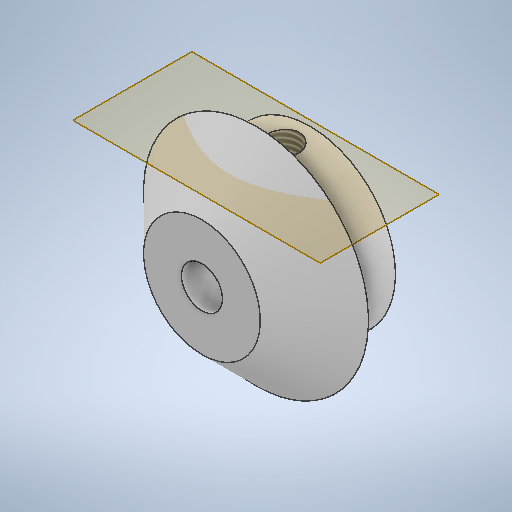
# Autodesk Inventor part: guide
Saved by Autodesk Inventor 2025.1 (Build 291241000, 241)
## iProperties
Created: 2025-03-11
Part Number: guide
Material: Generic
Document SubType Name: Modeling
Designer: santiago
Density: 1 g/cm^3
Appearance: Default
Author: santiago
Autodesk Inventor part; units mm, degrees
ref_plane "YZ Plane" through (0, 0, 0) normal (1, 0, 0) x (0, 1, 0)
ref_plane "XY Plane" through (0, 0, 0) normal (0, 0, 1) x (1, 0, 0)
sketch "Sketch1" plane through (0, 0, 0) normal (1, 0, 0) x (0, 1, 0)
  line L0 (0.0289, 5.9359) -> (3.5289, 5.9359)
  line L1 (0.0289, 5.9359) -> (0.0289, -4.0641)
  line L2 (-1.8711, 5.9359) -> (-1.8711, -4.0641) construction
  line L3 (6.0289, 0.9359) -> (8.5289, 0.9359)
  line L4 (3.5289, 5.9359) -> (8.5289, 0.9359)
  line L5 (0.0289, -4.0641) -> (6.0289, -4.0641)
  line L6 (6.0289, -4.0641) -> (6.0289, 0.9359)
  point P0 (0, 0)
  dimension "d0" = 3.5
  dimension "d3" = 10
  dimension "d4" = 1.9
  constraints: 14 end point, 3 horizontal, 2 vertical, 1 perpendicular
  measures "d0" distance of L0.start L0.end
  measures "d3" distance of L0.start L1.end
  measures "d4" distance between parallel lines of L1 L2
revolve "Revolution1" add sketch "Sketch1" angle 360 about axis through (0, -1.8711, 5.9359) along (0, 0, -1)
ref_plane "Work Plane1" through (0, 6.0289, -1.5641) normal (0, 1, 0) x (-1, 0, 0)
sketch "Sketch2" plane through (0, 6.0289, -1.5641) normal (0, 1, 0) x (-1, 0, 0)
  circle A0 centre (0, 0) radius 1.5
  point P0 (0, 1.5641)
  dimension "d6" = 3
  constraints: 1 centre point
  measures "d6" diameter of A0
extrude "Extrusion1" cut sketch "Sketch2" against normal up to surface round surface about axis through (0, -1.8711, 0.9359) along (0, 0, -1) radius 1.9 far side no
thread "Thread1" size "M3x0.5" class "6H" standard "ANSI Metric M Profile" full length
body "Solid1"
